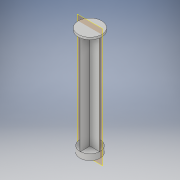
# Autodesk Inventor part: CH_01_0007_piston
Saved by Autodesk Inventor 2019 (Build 230136000, 136)
## iProperties
Created: 2022-02-23
Part Number: CH_01_0007_piston
Material: Generic
Document SubType Name: Modeling
Designer: Tomasz Krakowski
Density: 1 g/cm^3
Appearance: Default
Author: Tomasz Krakowski
Autodesk Inventor part; units mm, degrees
ref_plane "YZ Plane" through (0, 0, 0) normal (1, 0, 0) x (0, 1, 0)
ref_plane "XZ Plane" through (0, 0, 0) normal (0, 1, 0) x (-1, 0, 0)
sketch "Sketch1" plane through (0, 0, 0) normal (0, 1, 0) x (-1, 0, 0)
  circle A0 centre (0, 0) radius 14
  dimension "d0" = 28
  constraints: 1 centre point, 1 coincident
  measures "d0" diameter of A0
extrude "Extrusion1" add sketch "Sketch1" along normal blind 8.2
sketch "Sketch2" plane through (0, 8.2, 0) normal (0, 1, 0) x (1, 0, 0)
  line L0 (-13.5, -0.75) -> (-13.5, 0.75)
  line L1 (13.5, 0.75) -> (13.5, -0.75)
  line L2 (13.5, -0.75) -> (-13.5, 0.75) construction
  line L3 (-13.5, -0.75) -> (13.5, 0.75) construction
  line L4 (0.75, -13.5) -> (-0.75, -13.5)
  line L5 (-0.75, 13.5) -> (0.75, 13.5)
  line L6 (0.75, -13.5) -> (-0.75, 13.5) construction
  line L7 (-0.75, -13.5) -> (0.75, 13.5) construction
  line L8 (-0.75, -13.5) -> (-0.75, -0.75)
  line L9 (-0.75, 0.75) -> (-0.75, 13.5)
  line L10 (-13.5, 0.75) -> (-0.75, 0.75)
  line L11 (13.5, -0.75) -> (0.75, -0.75)
  line L12 (-0.75, -0.75) -> (-13.5, -0.75)
  line L13 (0.75, 13.5) -> (0.75, 0.75)
  line L14 (0.75, -0.75) -> (0.75, -13.5)
  line L15 (0.75, 0.75) -> (13.5, 0.75)
  point P0 (0, 0)
  dimension "d3" = 1.5
  dimension "d4" = 27
  dimension "d5" = 27
  constraints: 32 end point, 10 parallel, 5 perpendicular, 4 collinear, 4 midpoint, 3 horizontal
  measures "d3" distance between parallel lines of L14 L8
  measures "d4" distance between parallel lines of L1 L0
  measures "d5" distance between parallel lines of L5 L4
extrude "Extrusion2" add sketch "Sketch2" along normal blind 138
sketch "Sketch3" plane through (0, 146.2, 0) normal (0, 1, 0) x (1, 0, 0)
  circle A0 centre (0, 0) radius 16.25
  dimension "d8" = 32.5
  constraints: 1 centre point, 1 coincident
  measures "d8" diameter of A0
extrude "Extrusion3" add sketch "Sketch3" along normal blind 3
equation "\"d5\" = d4"
equation "\"d18\" = d17"
equation "\"d17\" = 2"
body "Solid1"
